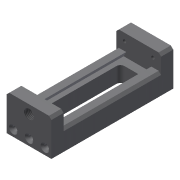
# Autodesk Inventor part: Base
Saved by Autodesk Inventor 2022 Beta2 (Build 260130000, 130) ContinuousBuild 0
## iProperties
Created: 2011-02-11
Part Number: Base
Material: Generic
Document SubType Name: Modeling
Designer: landrews
Density: 1 g/cm^3
Appearance: Light Gray
Author: landrews
Autodesk Inventor part; units mm, degrees
note: some values were not read from the file. Chosen so that the rebuilt part matches the saved one: direction of "Hole1".
ref_plane "YZ Plane" through (0, 0, 0) normal (1, 0, 0) x (0, 1, 0)
ref_plane "XZ Plane" through (0, 0, 0) normal (0, 1, 0) x (-1, 0, 0)
ref_plane "XY Plane" through (0, 0, 0) normal (0, 0, 1) x (1, 0, 0)
sketch "Sketch1" plane through (0, 0, -12.5) normal (0, 1, 0) x (-1, 0, 0)
  line L0 (-27.5, 12.5) -> (27.5, 12.5)
  line L1 (27.5, 12.5) -> (27.5, 37.5)
  line L2 (27.5, 37.5) -> (15.5, 37.5)
  line L3 (15.5, 37.5) -> (18.5, 31.5)
  line L4 (18.5, 31.5) -> (-18.5, 31.5)
  line L5 (-18.5, 31.5) -> (-15.5, 37.5)
  line L6 (-15.5, 37.5) -> (-27.5, 37.5)
  line L7 (-27.5, 37.5) -> (-27.5, 12.5)
  line L8 (0, 7.5) -> (0, 42.5) projected
  line L9 (-38.5, 12.5) -> (38.5, 12.5) projected
  point P0 (0, 12.5)
  point P1 (0, 12.5)
  dimension "Base_Width" = 55
  dimension "Base_Height" = 25
  dimension "Slider_Shelf" = 12
  dimension "d3" = 9
  dimension "d2" = 6
  constraints: 16 end point, 4 parallel, 2 equal length, 2 midpoint, 1 coincident, 1 collinear, 1 horizontal, 1 perpendicular, 1 other
  measures "Base_Width" distance of L0.start L0.end
  measures "Base_Height" distance of L0.end L1.end
  measures "Slider_Shelf" distance of L1.end L2.end
  measures "d3" horizontal distance of L1.end L3.end
  measures "d2" distance between parallel lines of L2 L4
extrude "Extrusion1" add sketch "Sketch1" along normal mid plane 120
sketch "Sketch4" plane through (-18.5, 60, 19) normal (0, 0, 1) x (1, 0, 0)
  line L0 (11, -110) -> (26, -110)
  line L1 (31, -105) -> (31, -15)
  line L2 (26, -10) -> (11, -10)
  line L3 (6, -15) -> (6, -105)
  arc A0 (6, -105) -> (11, -110) centre (11, -105) ccw
  arc A1 (26, -110) -> (31, -105) centre (26, -105) ccw
  arc A2 (31, -15) -> (26, -10) centre (26, -15) ccw
  arc A3 (11, -10) -> (6, -15) centre (11, -15) ccw
  line L4 (-20, -60) -> (57, -60) projected
  line L5 (18.5, 24) -> (18.5, -144) projected
  line L6 (-9, -120) -> (-9, 0) projected
  line L7 (37, 0) -> (0, 0) projected
  dimension "StopPlate_DP" = 5
  dimension "d25" = 100
  dimension "d26" = 25
  constraints: 8 end point, 8 point on circle, 8 tangent, 4 centre point, 3 equal radius, 2 parallel, 1 horizontal, 1 perpendicular, 2 other
  measures "StopPlate_DP" radius of A0
  measures "d25" distance between parallel lines of L0 L2
  measures "d26" distance between parallel lines of L1 L3
extrude "Extrusion2" cut sketch "Sketch4" against normal through all
sketch "Sketch6" plane through (0, -60, -12.5) normal (0, -1, 0) x (1, 0, 0)
  line L0 (27.5, 37.5) -> (27.5, 12.5) projected
  line L1 (-27.5, 12.5) -> (27.5, 12.5)
  line L2 (27.5, 12.5) -> (27.5, 57)
  line L3 (27.5, 57) -> (-27.5, 57)
  line L4 (-27.5, 57) -> (-27.5, 12.5)
  point P0 (0, 12.5)
  dimension "EndBlock_HT" = 44.5
  constraints: 8 end point, 2 parallel, 1 horizontal, 1 perpendicular, 1 point on line
  measures "EndBlock_HT" distance between parallel lines of L1 L3
extrude "Extrusion4" add sketch "Sketch6" along normal blind 15
mirror "Mirror1" about plane through (0, 0, 0) normal (0, 1, 0) of "Extrusion4"
sketch "Sketch7" plane through (0, -75, -12.5) normal (0, -1, 0) x (1, 0, 0)
  line L0 (-27.5, 57) -> (27.5, 57) projected
  line L1 (0, 65.9) -> (0, 3.6) projected
  point P0 (0, 12.5)
  point P1 (0, 46.5)
  dimension "d39" = 10.5
  constraints: 1 point on line
  measures "d39" distance from line of point (0, 46.5) L0
hole "Hole1" at (0, -75, 34) direction (0, 1, 0) diameter 12 depth 75
sketch "Sketch14" plane through (0, -75, -12.5) normal (0, -1, 0) x (1, 0, 0)
  line L0 (27.5, 12.5) -> (-27.5, 12.5) projected
  line L1 (0, 65.9) -> (0, 3.6) projected
  point P0 (0, 12.5)
  point P1 (0, 20.5)
  dimension "d83" = 8
  constraints: 1 point on line
  measures "d83" distance from line of L0 point (0, 20.5)
hole "Hole5" at (0, -75, 8) direction (0, 1, 0) diameter 6 depth 15 tip angle 118 countersink diameter 10.4 countersink angle 90
sketch "Sketch9" plane through (0, -60, -12.5) normal (0, -1, 0) x (1, 0, 0)
  circle A0 centre (0, 20.5) radius 5.2 projected
  point P0 (0, 12.5)
  constraints: 1 coincident
hole "Hole3" at (0, -60, 8) direction (0, 1, 0) diameter 4.134 depth 8 tip angle 118 thread size "M5x0.8" class "6H" standard "ANSI Metric M Profile"
pattern_linear "Rectangular Pattern2" count 3 spacing 19.5 along (-1, 0, 0) of "Hole3", "Hole5" first direction both ways yes
mirror "Mirror2" about plane through (0, 0, 0) normal (0, 1, 0) of "Hole3", "Rectangular Pattern2", "Hole5"
sketch "Sketch11" plane through (-27.5, 60, 44.5) normal (0, -1, 0) x (1, 0, 0)
  line L0 (0, 0) -> (55, 0) projected
  line L1 (0, -44.5) -> (0, 0) projected
  line L2 (55, 0) -> (55, -44.5) projected
  point P0 (27.5, -44.5)
  point P1 (10, -9)
  point P2 (45, -9)
  dimension "d103" = 9
  dimension "d104" = 10
  dimension "d105" = 10
  constraints: 1 horizontal alignment
  measures "d103" distance from line of L0 point (10, -9)
  measures "d104" distance from line of L1 point (10, -9)
  measures "d105" distance from line of L2 point (45, -9)
hole "Hole6" at (-17.5, 60, 35.5) at (17.5, 60, 35.5) direction (0, 1, 0) diameter 4.134 depth 10 tip angle 118 thread size "M5x0.8" class "6H" standard "ANSI Metric M Profile"
thread "Thread1" size "M12x1.75" class "6H" standard "ANSI Metric M Profile" full length
chamfer "Chamfer1" distance 3 angle 45 6 edges at (-27.5, -67.5, 44.5) (27.5, -67.5, 44.5) (27.5, 67.5, 44.5) (-27.5, 67.5, 44.5) (27.5, 0, 25) (-27.5, 0, 25)
equation "\"d89\" = EndBlock_DP"
equation "\"d104\" = d105"
equation "\"EndBlock_DP\" = 15"
body "Solid1"
